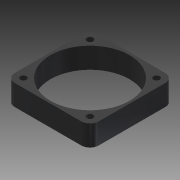
# Autodesk Inventor part: Ventilador
Saved by Autodesk Inventor 2014 (Build 180170000, 170)
## iProperties
Created: 2014-09-11
Part Number: Ventilador
Material: Rubber, Silicone
Document SubType Name: Modeling
Designer: Rubén
Density: 1.25 g/cm^3
Appearance: Rubber - Black - Version 1.1
Mass: 21.7922 g
Surface Area: 52.8102 cm^2
Volume: 17.4337 cm^3
Author: Rubén
Autodesk Inventor part; units mm, degrees
ref_plane "YZ Plane" through (0, 0, 0) normal (1, 0, 0) x (0, 1, 0)
ref_plane "XZ Plane" through (0, 0, 0) normal (0, 1, 0) x (-1, 0, 0)
ref_plane "XY Plane" through (0, 0, 0) normal (0, 0, 1) x (1, 0, 0)
sketch "Sketch1" plane through (0, 0, 0) normal (0, 1, 0) x (-1, 0, 0)
  line L0 (4.175, 0) -> (36.175, 0)
  line L1 (40.35, 4.175) -> (40.35, 36.175)
  line L2 (36.175, 40.35) -> (4.175, 40.35)
  line L3 (0, 36.175) -> (0, 4.175)
  circle A0 centre (4.175, 4.175) radius 1.5
  circle A1 centre (36.175, 4.175) radius 1.5
  circle A2 centre (4.175, 36.175) radius 1.5
  circle A3 centre (36.175, 36.175) radius 1.5
  arc A4 (4.175, 40.35) -> (0, 36.175) centre (4.175, 36.175) ccw
  arc A5 (40.35, 36.175) -> (36.175, 40.35) centre (36.175, 36.175) ccw
  arc A6 (36.175, 0) -> (40.35, 4.175) centre (36.175, 4.175) ccw
  arc A7 (0, 4.175) -> (4.175, 0) centre (4.175, 4.175) ccw
  circle A8 centre (20.175, 20.175) radius 19
  point P0 (0, 0)
  point P1 (40.35, 0)
  point P2 (40.35, 40.35)
  dimension "d0" = 40.35
  dimension "d1" = 40.35
  dimension "d2" = 3
  dimension "d5" = 32
  dimension "d8" = 32
  dimension "d12" = 4.175
  dimension "d15" = 38
  dimension "d16" = 20.175
  dimension "d17" = 20.175
  constraints: 9 centre point, 8 end point, 8 point on circle, 8 tangent, 6 point on line, 3 equal radius, 2 horizontal, 2 perpendicular, 1 coincident, 1 parallel, 1 vertical, 6 other
  measures "d0" distance of point (0, 0) point (40.35, 0)
  measures "d1" distance of point (40.35, 0) point (40.35, 40.35)
  measures "d2" diameter of A0
  measures "d5" distance of A0.centre A1.centre
  measures "d8" distance of A0.centre A2.centre
  measures "d12" radius of A4
  measures "d15" diameter of A8
  measures "d16" distance from line of A8.centre L1
  measures "d17" distance from line of A8.centre L2
extrude "Extrusion2" add sketch "Sketch1" along normal blind 10
body "Solid2"
